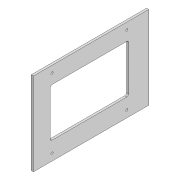
# Autodesk Inventor part: BREEZE-M06
Saved by Autodesk Inventor 2020 (Build 240168000, 168)
## iProperties
Created: 2020-04-12
Part Number: BREEZE-M06
Material: Generic
Description: SCREEN PANEL
Document SubType Name: Modeling
Designer: John K
Density: 1 g/cm^3
Appearance: Default
Author: John K
Autodesk Inventor part; units mm, degrees
ref_plane "YZ Plane" through (0, 0, 0) normal (1, 0, 0) x (0, 1, 0)
ref_plane "XZ Plane" through (0, 0, 0) normal (0, 1, 0) x (-1, 0, 0)
ref_plane "XY Plane" through (0, 0, 0) normal (0, 0, 1) x (1, 0, 0)
sketch "Face" plane through (0, 0, 0) normal (0, 0, 1) x (1, 0, 0)
  line L0 (38.5, 208.87) -> (135.1, 208.87)
  arc A0 (38.5, 208.87) -> (34.5, 204.87) centre (38.5, 204.87) ccw
  circle A1 centre (10, 204.87) radius 2.6
  line L1 (175.25, 245.25) -> (-4.75, 245.25)
  line L2 (139.1, 204.87) -> (139.1, 42.67)
  line L3 (34.5, 42.67) -> (34.5, 204.87)
  line L4 (175.25, -4.75) -> (175.25, 245.25)
  line L5 (-4.75, 245.25) -> (-4.75, -4.75)
  circle A2 centre (160.5, 42.67) radius 2.6
  arc A3 (135.1, 38.67) -> (139.1, 42.67) centre (135.1, 42.67) ccw
  arc A4 (34.5, 42.67) -> (38.5, 38.67) centre (38.5, 42.67) ccw
  circle A5 centre (10, 42.67) radius 2.6
  line L6 (-4.75, -4.75) -> (175.25, -4.75)
  line L7 (135.1, 38.67) -> (38.5, 38.67)
  arc A6 (139.1, 204.87) -> (135.1, 208.87) centre (135.1, 204.87) ccw
  circle A7 centre (160.5, 204.87) radius 2.6
  point P0 (84.3959, 120.382)
  point P1 (0, 0)
sketch "Sketch1" plane through (0, 0, 0) normal (1, 0, 0) x (0, 1, 0)
  line L0 (-46.75, 88.62) -> (49.85, 88.62)
  arc A0 (-46.75, 88.62) -> (-50.75, 84.62) centre (-46.75, 84.62) ccw
  circle A1 centre (-75.25, 84.62) radius 2.6
  line L1 (90, 125) -> (-90, 125)
  line L2 (53.85, 84.62) -> (53.85, -77.58)
  line L3 (-50.75, -77.58) -> (-50.75, 84.62)
  line L4 (90, -125) -> (90, 125)
  line L5 (-90, 125) -> (-90, -125)
  circle A2 centre (75.25, -77.58) radius 2.6
  arc A3 (49.85, -81.58) -> (53.85, -77.58) centre (49.85, -77.58) ccw
  arc A4 (-50.75, -77.58) -> (-46.75, -81.58) centre (-46.75, -77.58) ccw
  circle A5 centre (-75.25, -77.58) radius 2.6
  line L6 (-90, -125) -> (90, -125)
  line L7 (49.85, -81.58) -> (-46.75, -81.58)
  arc A6 (53.85, 84.62) -> (49.85, 88.62) centre (49.85, 84.62) ccw
  circle A7 centre (75.25, 84.62) radius 2.6
  point P0 (0, 0)
  point P1 (0, 125)
  point P2 (90, 0)
  constraints: 1 horizontal alignment, 1 vertical alignment, 2 other
extrude "Extrusion1" add sketch "Sketch1" along normal mid plane 4.75
body "Solid1"
